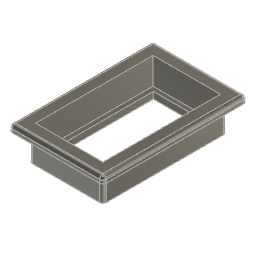
Spin Insert v2 (Autodesk Fusion 360 design; units mm, degrees)
Autodesk Fusion 360 part; units mm, degrees
sketch "Sketch1" plane through (0, 0, 0) normal (0, 0, 1) x (1, 0, 0)
  line L0 (5.55, 9.3) -> (-5.55, 9.3)
  line L1 (-5.55, 9.3) -> (-5.55, -9.3)
  line L2 (-5.55, -9.3) -> (5.55, -9.3)
  line L3 (5.55, -9.3) -> (5.55, 9.3)
  line L4 (5.55, 9.3) -> (-5.55, -9.3) construction
  line L5 (-5.55, 9.3) -> (5.55, -9.3) construction
  line L6 (7.05, -10.8) -> (-7.05, -10.8)
  line L7 (-7.05, -10.8) -> (-7.05, 10.8)
  line L8 (-7.05, 10.8) -> (7.05, 10.8)
  line L9 (7.05, 10.8) -> (7.05, -10.8)
  line L10 (7.05, -10.8) -> (-7.05, 10.8) construction
  line L11 (-7.05, -10.8) -> (7.05, 10.8) construction
  line L12 (5.05, -8.8) -> (-5.05, -8.8)
  line L13 (-5.05, -8.8) -> (-5.05, 8.8)
  line L14 (-5.05, 8.8) -> (5.05, 8.8)
  line L15 (5.05, 8.8) -> (5.05, -8.8)
  line L16 (5.05, -8.8) -> (-5.05, 8.8) construction
  line L17 (-5.05, -8.8) -> (5.05, 8.8) construction
  dimension "d1" = 11.1
  dimension "d2" = 18.6
  dimension "d3" = 14.1
  dimension "d4" = 21.6
  dimension "d5" = 10.1
  dimension "d6" = 17.6
  constraint horizontal L0
  constraint perpendicular L0 L1
  constraint parallel L0 L2
  constraint parallel L1 L3
  constraint coincident L4 origin
  constraint coincident L5 origin
  constraint horizontal L6
  constraint perpendicular L6 L7
  constraint parallel L6 L8
  constraint parallel L7 L9
  constraint coincident L10 origin
  constraint coincident L11 origin
  constraint horizontal L12
  constraint perpendicular L12 L13
  constraint parallel L12 L14
  constraint parallel L13 L15
  constraint coincident L16 origin
  constraint coincident L17 origin
  measures "d1" distance of L1.end L2.end
  measures "d2" distance of L0.end L1.end
  measures "d3" distance of L7.end L8.end
  measures "d4" distance of L6.end L7.end
  measures "d5" distance of L13.end L14.end
  measures "d6" distance of L12.end L13.end
extrude "Extrude1" add sketch "Sketch1" along normal blind 1 contours L0 L1 L2 L3 | L6 L7 L8 L9
extrude "Extrude2" add sketch "Sketch1" against normal blind 3 contours L0 L1 L2 L3
sketch "Sketch2" plane through (0, 0, -3) normal (0, 0, -1) x (1, 0, 0)
  line L0 (5.05, -8.8) -> (-5.05, -8.8)
  line L1 (-5.05, -8.8) -> (-5.05, 8.8)
  line L2 (-5.05, 8.8) -> (5.05, 8.8)
  line L3 (5.05, 8.8) -> (5.05, -8.8)
  line L4 (5.55, -9.3) -> (5.55, 9.3)
  line L5 (5.55, 9.3) -> (-5.55, 9.3)
  line L6 (-5.55, 9.3) -> (-5.55, -9.3)
  line L7 (-5.55, -9.3) -> (5.55, -9.3)
  line L8 (5.55, -9.3) -> (-5.55, -9.3)
  line L9 (-5.55, -9.3) -> (-5.55, 9.3)
  line L10 (-5.55, 9.3) -> (5.55, 9.3)
  line L11 (5.55, 9.3) -> (5.55, -9.3)
  line L12 (5.55, -9.3) -> (-5.55, 9.3) construction
  line L13 (-5.55, -9.3) -> (5.55, 9.3) construction
  line L14 (4.35, -8.15) -> (-4.35, -8.15)
  line L15 (-4.35, -8.15) -> (-4.35, 8.15)
  line L16 (-4.35, 8.15) -> (4.35, 8.15)
  line L17 (4.35, 8.15) -> (4.35, -8.15)
  line L18 (4.35, -8.15) -> (-4.35, 8.15) construction
  line L19 (-4.35, -8.15) -> (4.35, 8.15) construction
  dimension "d11" = 8.7
  dimension "d12" = 16.3
  constraint horizontal L8
  constraint perpendicular L8 L9
  constraint parallel L8 L10
  constraint parallel L9 L11
  constraint coincident L4.start L7.end
  constraint coincident L12 origin
  constraint coincident L13 origin
  constraint horizontal L14
  constraint perpendicular L14 L15
  constraint parallel L14 L16
  constraint parallel L15 L17
  constraint coincident L18 origin
  constraint coincident L19 origin
  measures "d11" distance of L15.end L16.end
  measures "d12" distance of L14.end L15.end
extrude "Extrude3" add sketch "Sketch2" along normal blind 1 contours L0 L1 L2 L3 | L4 L5 L6 L7 L8 L9 L10 L11
fillet "Fillet1" radius 0.5 8 edges at (-7.05, -10.8, 0.5) (7.05, -10.8, 0.5) (-5.55, -9.3, -2) (5.55, -9.3, -2) (-5.55, 9.3, -2) (-7.05, 10.8, 0.5) (5.55, 9.3, -2) (7.05, 10.8, 0.5)
fillet "Fillet2" radius 0.5 8 edges at (6.9036, -10.6536, 1) (7.05, 0, 1) (6.9036, 10.6536, 1) (0, 10.8, 1) (-6.9036, 10.6536, 1) (-7.05, 0, 1) (-6.9036, -10.6536, 1) (0, -10.8, 1)
